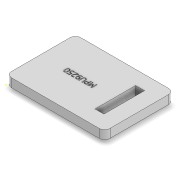
# Autodesk Inventor part: Gyro_box_Top
Saved by Autodesk Inventor 2020 (Build 240168000, 168)
## iProperties
Created: 2019-08-08
Part Number: Gyro_box_Top
Material: Generic
Document SubType Name: Modeling
Designer: chitl
Density: 1 g/cm^3
Appearance: Default
Author: chitl
Autodesk Inventor part; units mm, degrees
ref_plane "YZ Plane" through (0, 0, 0) normal (1, 0, 0) x (0, 1, 0)
ref_plane "XZ Plane" through (0, 0, 0) normal (0, 1, 0) x (-1, 0, 0)
ref_plane "XY Plane" through (0, 0, 0) normal (0, 0, 1) x (1, 0, 0)
sketch "Sketch1" plane through (0, 0, 0) normal (0, 1, 0) x (-1, 0, 0)
  line L0 (0, 0) -> (-56.9976, 0)
  line L1 (-56.9976, 0) -> (-56.9976, -40.1066)
  line L2 (-56.9976, -40.1066) -> (0, -40.1066)
  line L3 (0, -40.1066) -> (0, 0)
  dimension "d0" = 40.1066
  dimension "d1" = 56.9976
  constraints: 8 end point, 2 parallel, 1 horizontal, 1 perpendicular
  measures "d0" distance of L2.end L0.start
  measures "d1" distance between parallel lines of L1 L3
extrude "Extrusion1" add sketch "Sketch1" along normal blind 5
fillet "Fillet1" radius 3.175 2 edges at (0, 2.5, 0) (0, 2.5, -40.1066)
fillet "Fillet2" radius 3.175 2 edges at (56.9976, 2.5, 0) (56.9976, 2.5, -40.1066)
sketch "Sketch2" plane through (0, 0, 0) normal (0, -1, 0) x (1, 0, 0)
  point P0 (0, 0)
sketch "Sketch3" plane through (0, 0, 0) normal (0, -1, 0) x (1, 0, 0)
  arc A0 (53.8226, -40.1066) -> (56.9976, -36.9316) centre (53.8226, -36.9316) ccw projected
  line L0 (56.9976, -3.175) -> (56.9976, -36.9316) projected
  arc A1 (56.9976, -3.175) -> (53.8226, 0) centre (53.8226, -3.175) ccw projected
  line L1 (3.175, 0) -> (53.8226, 0) projected
  arc A2 (3.175, 0) -> (0, -3.175) centre (3.175, -3.175) ccw projected
  line L2 (0, -36.9316) -> (0, -3.175) projected
  arc A3 (0, -36.9316) -> (3.175, -40.1066) centre (3.175, -36.9316) ccw projected
  line L3 (53.8226, -40.1066) -> (3.175, -40.1066) projected
  arc A4 (53.8734, -3.175) -> (53.8226, -3.1242) centre (53.8226, -3.175) ccw
  line L4 (53.8734, -3.175) -> (53.8734, -36.9316)
  arc A5 (53.8226, -36.9824) -> (53.8734, -36.9316) centre (53.8226, -36.9316) ccw
  line L5 (53.8226, -36.9824) -> (3.175, -36.9824)
  arc A6 (3.1242, -36.9316) -> (3.175, -36.9824) centre (3.175, -36.9316) ccw
  line L6 (3.1242, -36.9316) -> (3.1242, -3.175)
  arc A7 (3.175, -3.1242) -> (3.1242, -3.175) centre (3.175, -3.175) ccw
  line L7 (3.175, -3.1242) -> (53.8226, -3.1242)
  point P0 (0, 0)
  dimension "d6" = 3.1242
  constraints: 8 end point, 8 point on circle, 4 centre point, 7 other
  measures "d6" distance between parallel lines of L1 L7
extrude "Extrusion2" add sketch "Sketch3" along normal blind 2 contours L4 A5 L5 A6 L6 A7 L7 A4
sketch "Sketch4" plane through (0, 5, 0) normal (0, 1, 0) x (1, 0, 0)
  line L0 (42.9327, 8.4905) -> (48.1076, 8.4905)
  line L1 (48.1076, 8.4905) -> (48.1076, 31.9976)
  line L2 (48.1076, 31.9976) -> (42.9327, 31.9976)
  line L3 (42.9327, 31.9976) -> (42.9327, 8.4905)
  line L4 (56.9976, 3.175) -> (56.9976, 36.9316) projected
  point P0 (0, 0)
  dimension "d9" = 8.89
  constraints: 8 end point, 2 parallel, 1 horizontal, 1 perpendicular
  measures "d9" distance between parallel lines of L1 L4
extrude "Extrusion3" cut sketch "Sketch4" against normal blind 20.225
sketch "Sketch5" plane through (0, 5, 0) normal (0, 1, 0) x (1, 0, 0)
  line L0 (31.7516, 18.1072) -> (19.4886, 18.1072) construction
  line L1 (19.4886, 18.1072) -> (19.4886, 46.8549) construction
  line L2 (19.4886, 46.8549) -> (31.7516, 46.8549) construction
  line L3 (31.7516, 46.8549) -> (31.7516, 18.1072) construction
  line L4 (28.8296, 21.2194) -> (29.2346, 21.2194)
  line L5 (29.2346, 21.2194) -> (29.2346, 18.5938)
  line L6 (29.2346, 18.5938) -> (30.03, 20.3796)
  line L7 (30.03, 20.3796) -> (30.277, 20.3796)
  line L8 (30.277, 20.3796) -> (31.0649, 18.5938)
  line L9 (31.0649, 18.5938) -> (31.0649, 21.2194)
  line L10 (31.0649, 21.2194) -> (31.4428, 21.2194)
  line L11 (31.4428, 21.2194) -> (31.4428, 18.1714)
  line L12 (31.4428, 18.1714) -> (30.8896, 18.1714)
  line L13 (30.8896, 18.1714) -> (30.1288, 19.8683)
  line L14 (30.1288, 19.8683) -> (29.3927, 18.1714)
  line L15 (29.3927, 18.1714) -> (28.8296, 18.1714)
  line L16 (28.8296, 18.1714) -> (28.8296, 21.2194)
  spline S0 degree 2 poles (26.2855, 19.0903) (26.2855, 19.2879) (26.4262, 19.6436) (26.5522, 19.7671) knots 0 0 0 1 2 2 2
  spline S1 degree 2 poles (26.5522, 19.7671) (26.7103, 19.9227) (27.1376, 20.0832) (27.4636, 20.0832) knots 0 0 0 1 2 2 2
  line L17 (27.4636, 20.0832) -> (27.807, 20.0832)
  line L18 (27.807, 20.0832) -> (27.807, 21.2194)
  line L19 (27.807, 21.2194) -> (28.2121, 21.2194)
  line L20 (28.2121, 21.2194) -> (28.2121, 18.1714)
  line L21 (28.2121, 18.1714) -> (27.4464, 18.1714)
  spline S2 degree 2 poles (27.4464, 18.1714) (27.1747, 18.1714) (26.7943, 18.2604) (26.6485, 18.3616) knots 0 0 0 1 2 2 2
  spline S3 degree 2 poles (26.6485, 18.3616) (26.4781, 18.4777) (26.2855, 18.8359) (26.2855, 19.0903) knots 0 0 0 1 2 2 2
  spline S4 degree 2 poles (26.7078, 19.1026) (26.7078, 18.9445) (26.8165, 18.7124) (26.9277, 18.6383) knots 0 0 0 1 2 2 2
  spline S5 degree 2 poles (26.9277, 18.6383) (27.024, 18.574) (27.2809, 18.5222) (27.4711, 18.5222) knots 0 0 0 1 2 2 2
  line L22 (27.4711, 18.5222) -> (27.807, 18.5222)
  line L23 (27.807, 18.5222) -> (27.807, 19.7374)
  line L24 (27.807, 19.7374) -> (27.5303, 19.7374)
  spline S6 degree 2 poles (27.5303, 19.7374) (27.2833, 19.7374) (26.9795, 19.6584) (26.8807, 19.5546) knots 0 0 0 1 2 2 2
  spline S7 degree 2 poles (26.8807, 19.5546) (26.7893, 19.4633) (26.7078, 19.2484) (26.7078, 19.1026) knots 0 0 0 1 2 2 2
  spline S8 degree 2 poles (24.8356, 21.2837) (25.1048, 21.2837) (25.5049, 21.1429) (25.6457, 21.0021) knots 0 0 0 1 2 2 2
  spline S9 degree 2 poles (25.6457, 21.0021) (25.8063, 20.844) (25.9372, 20.3994) (25.9372, 20.0733) knots 0 0 0 1 2 2 2
  line L25 (25.9372, 20.0733) -> (25.9372, 18.1714)
  line L26 (25.9372, 18.1714) -> (25.5321, 18.1714)
  line L27 (25.5321, 18.1714) -> (25.5321, 20.0733)
  spline S10 degree 2 poles (25.5321, 20.0733) (25.5321, 20.2858) (25.4778, 20.5723) (25.4012, 20.6884) knots 0 0 0 1 2 2 2
  spline S11 degree 2 poles (25.4012, 20.6884) (25.3197, 20.8119) (25.0381, 20.9379) (24.8356, 20.9379) knots 0 0 0 1 2 2 2
  spline S12 degree 2 poles (24.8356, 20.9379) (24.6454, 20.9379) (24.349, 20.8119) (24.2674, 20.6884) knots 0 0 0 1 2 2 2
  spline S13 degree 2 poles (24.2674, 20.6884) (24.1909, 20.5723) (24.1365, 20.2882) (24.1365, 20.0832) knots 0 0 0 1 2 2 2
  line L28 (24.1365, 20.0832) -> (24.1365, 18.1714)
  line L29 (24.1365, 18.1714) -> (23.7315, 18.1714)
  line L30 (23.7315, 18.1714) -> (23.7315, 20.0733)
  spline S14 degree 2 poles (23.7315, 20.0733) (23.7315, 20.392) (23.8599, 20.8465) (24.0229, 21.0021) knots 0 0 0 1 2 2 2
  spline S15 degree 2 poles (24.0229, 21.0021) (24.1686, 21.1453) (24.554, 21.2837) (24.8356, 21.2837) knots 0 0 0 1 2 2 2
  spline S16 degree 2 poles (23.3214, 19.1619) (23.3214, 18.9273) (23.1683, 18.537) (23.0349, 18.3962) knots 0 0 0 1 2 2 2
  spline S17 degree 2 poles (23.0349, 18.3962) (22.9089, 18.2604) (22.5409, 18.1097) (22.3532, 18.1097) knots 0 0 0 1 2 2 2
  spline S18 degree 2 poles (22.3532, 18.1097) (22.1432, 18.1097) (21.8024, 18.2505) (21.6764, 18.3839) knots 0 0 0 1 2 2 2
  spline S19 degree 2 poles (21.6764, 18.3839) (21.5183, 18.5518) (21.3454, 19.0952) (21.3454, 19.5127) knots 0 0 0 1 2 2 2
  spline S20 degree 2 poles (21.3454, 19.5127) (21.3454, 19.8906) (21.5158, 20.5673) (21.6813, 20.7921) knots 0 0 0 1 2 2 2
  spline S21 degree 2 poles (21.6813, 20.7921) (21.8567, 21.0292) (22.3507, 21.2787) (22.7113, 21.2787) knots 0 0 0 1 2 2 2
  spline S22 degree 2 poles (22.7113, 21.2787) (22.7928, 21.2787) (22.9781, 21.2614) (23.0571, 21.2367) knots 0 0 0 1 2 2 2
  line L31 (23.0571, 21.2367) -> (23.0571, 20.844)
  line L32 (23.0571, 20.844) -> (23.0374, 20.844)
  spline S23 degree 2 poles (23.0374, 20.844) (22.9855, 20.8736) (22.7681, 20.9255) (22.657, 20.9255) knots 0 0 0 1 2 2 2
  spline S24 degree 2 poles (22.657, 20.9255) (22.2569, 20.9255) (21.7999, 20.3969) (21.7678, 19.9079) knots 0 0 0 1 2 2 2
  spline S25 degree 2 poles (21.7678, 19.9079) (21.9308, 20.019) (22.2272, 20.1203) (22.4026, 20.1203) knots 0 0 0 1 2 2 2
  spline S26 degree 2 poles (22.4026, 20.1203) (22.5705, 20.1203) (22.8497, 20.0462) (22.9904, 19.94) knots 0 0 0 1 2 2 2
  spline S27 degree 2 poles (22.9904, 19.94) (23.1535, 19.814) (23.3214, 19.4311) (23.3214, 19.1619) knots 0 0 0 1 2 2 2
  spline S28 degree 2 poles (21.7579, 19.4213) (21.7579, 19.1125) (21.8715, 18.7222) (21.9728, 18.616) knots 0 0 0 1 2 2 2
  spline S29 degree 2 poles (21.9728, 18.616) (22.0617, 18.5172) (22.247, 18.4431) (22.3557, 18.4431) knots 0 0 0 1 2 2 2
  spline S30 degree 2 poles (22.3557, 18.4431) (22.6076, 18.4431) (22.9065, 18.8038) (22.9065, 19.1446) knots 0 0 0 1 2 2 2
  spline S31 degree 2 poles (22.9065, 19.1446) (22.9065, 19.3373) (22.8077, 19.5868) (22.699, 19.6757) knots 0 0 0 1 2 2 2
  spline S32 degree 2 poles (22.699, 19.6757) (22.6199, 19.7399) (22.4248, 19.7819) (22.3112, 19.7819) knots 0 0 0 1 2 2 2
  spline S33 degree 2 poles (22.3112, 19.7819) (22.1803, 19.7819) (21.8789, 19.6905) (21.7653, 19.6139) knots 0 0 0 1 2 2 2
  spline S34 degree 2 poles (21.7653, 19.6139) (21.7629, 19.5843) (21.7579, 19.483) (21.7579, 19.4213) knots 0 0 0 1 2 2 2
  line L33 (19.0705, 21.2194) -> (20.9502, 21.2194)
  line L34 (20.9502, 21.2194) -> (20.9502, 20.7872)
  spline S35 degree 2 poles (20.9502, 20.7872) (20.7477, 20.597) (20.3871, 20.2438) (20.2142, 20.0536) knots 0 0 0 1 2 2 2
  spline S36 degree 2 poles (20.2142, 20.0536) (19.8659, 19.6707) (19.6115, 19.2113) (19.6115, 18.9668) knots 0 0 0 1 2 2 2
  spline S37 degree 2 poles (19.6115, 18.9668) (19.6115, 18.8383) (19.6905, 18.6457) (19.7621, 18.5839) knots 0 0 0 1 2 2 2
  spline S38 degree 2 poles (19.7621, 18.5839) (19.8338, 18.5222) (20.0215, 18.4604) (20.1351, 18.4604) knots 0 0 0 1 2 2 2
  spline S39 degree 2 poles (20.1351, 18.4604) (20.2438, 18.4604) (20.4661, 18.5148) (20.5674, 18.5568) knots 0 0 0 1 2 2 2
  spline S40 degree 2 poles (20.5674, 18.5568) (20.6538, 18.5913) (20.8144, 18.6901) (20.8638, 18.7247) knots 0 0 0 1 2 2 2
  line L35 (20.8638, 18.7247) -> (20.886, 18.7247)
  line L36 (20.886, 18.7247) -> (20.886, 18.29)
  spline S41 degree 2 poles (20.886, 18.29) (20.76, 18.2282) (20.308, 18.1072) (20.1055, 18.1072) knots 0 0 0 1 2 2 2
  spline S42 degree 2 poles (20.1055, 18.1072) (19.6782, 18.1072) (19.1965, 18.5592) (19.1965, 18.9445) knots 0 0 0 1 2 2 2
  spline S43 degree 2 poles (19.1965, 18.9445) (19.1965, 19.1249) (19.2805, 19.4262) (19.3546, 19.5546) knots 0 0 0 1 2 2 2
  spline S44 degree 2 poles (19.3546, 19.5546) (19.4287, 19.688) (19.6436, 19.9498) (19.7621, 20.0758) knots 0 0 0 1 2 2 2
  spline S45 degree 2 poles (19.7621, 20.0758) (19.9548, 20.2858) (20.4266, 20.7353) (20.5674, 20.8662) knots 0 0 0 1 2 2 2
  line L37 (20.5674, 20.8662) -> (19.0705, 20.8662)
  line L38 (19.0705, 20.8662) -> (19.0705, 21.2194)
  spline S46 degree 2 poles (16.8154, 20.2512) (16.8154, 20.471) (16.9562, 20.8465) (17.0846, 20.9848) knots 0 0 0 1 2 2 2
  spline S47 degree 2 poles (17.0846, 20.9848) (17.2131, 21.1231) (17.5959, 21.2837) (17.8331, 21.2837) knots 0 0 0 1 2 2 2
  spline S48 degree 2 poles (17.8331, 21.2837) (18.0504, 21.2837) (18.4753, 21.1873) (18.6309, 21.1108) knots 0 0 0 1 2 2 2
  line L39 (18.6309, 21.1108) -> (18.6309, 20.6785)
  line L40 (18.6309, 20.6785) -> (18.6012, 20.6785)
  spline S49 degree 2 poles (18.6012, 20.6785) (18.5543, 20.7131) (18.3789, 20.802) (18.2727, 20.8415) knots 0 0 0 1 2 2 2
  spline S50 degree 2 poles (18.2727, 20.8415) (18.1517, 20.8835) (17.9516, 20.9304) (17.8256, 20.9304) knots 0 0 0 1 2 2 2
  spline S51 degree 2 poles (17.8256, 20.9304) (17.7021, 20.9304) (17.47, 20.8415) (17.386, 20.7452) knots 0 0 0 1 2 2 2
  spline S52 degree 2 poles (17.386, 20.7452) (17.3094, 20.6538) (17.2304, 20.4117) (17.2304, 20.2487) knots 0 0 0 1 2 2 2
  spline S53 degree 2 poles (17.2304, 20.2487) (17.2304, 20.0857) (17.3193, 19.8782) (17.4033, 19.8091) knots 0 0 0 1 2 2 2
  spline S54 degree 2 poles (17.4033, 19.8091) (17.4897, 19.7325) (17.7466, 19.6683) (17.9022, 19.6683) knots 0 0 0 1 2 2 2
  spline S55 degree 2 poles (17.9022, 19.6683) (18.0702, 19.6683) (18.4036, 19.7201) (18.5049, 19.7424) knots 0 0 0 1 2 2 2
  line L41 (18.5049, 19.7424) -> (18.5049, 18.1714)
  line L42 (18.5049, 18.1714) -> (16.8327, 18.1714)
  line L43 (16.8327, 18.1714) -> (16.8327, 18.5296)
  line L44 (16.8327, 18.5296) -> (18.1122, 18.5296)
  line L45 (18.1122, 18.5296) -> (18.1122, 19.3422)
  spline S56 degree 2 poles (18.1122, 19.3422) (18.0381, 19.3323) (17.8948, 19.3249) (17.8355, 19.3249) knots 0 0 0 1 2 2 2
  spline S57 degree 2 poles (17.8355, 19.3249) (17.6009, 19.3249) (17.2773, 19.4015) (17.1291, 19.5151) knots 0 0 0 1 2 2 2
  spline S58 degree 2 poles (17.1291, 19.5151) (16.9784, 19.6287) (16.8154, 19.9745) (16.8154, 20.2512) knots 0 0 0 1 2 2 2
  spline S59 degree 2 poles (14.4788, 19.6954) (14.4788, 20.5155) (14.9555, 21.2837) (15.452, 21.2837) knots 0 0 0 1 2 2 2
  spline S60 degree 2 poles (15.452, 21.2837) (15.9558, 21.2837) (16.4276, 20.5007) (16.4276, 19.6979) knots 0 0 0 1 2 2 2
  spline S61 degree 2 poles (16.4276, 19.6979) (16.4276, 18.8729) (15.9509, 18.1097) (15.452, 18.1097) knots 0 0 0 1 2 2 2
  spline S62 degree 2 poles (15.452, 18.1097) (14.9505, 18.1097) (14.4788, 18.9001) (14.4788, 19.6954) knots 0 0 0 1 2 2 2
  spline S63 degree 2 poles (15.0024, 20.6242) (14.9431, 20.4735) (14.8937, 20.0091) (14.8937, 19.6954) knots 0 0 0 1 2 2 2
  spline S64 degree 2 poles (14.8937, 19.6954) (14.8937, 19.3817) (14.9431, 18.9198) (15.0049, 18.7642) knots 0 0 0 1 2 2 2
  spline S65 degree 2 poles (15.0049, 18.7642) (15.0666, 18.6086) (15.2815, 18.4481) (15.452, 18.4481) knots 0 0 0 1 2 2 2
  spline S66 degree 2 poles (15.452, 18.4481) (15.6224, 18.4481) (15.8422, 18.6086) (15.9064, 18.7692) knots 0 0 0 1 2 2 2
  spline S67 degree 2 poles (15.9064, 18.7692) (15.9682, 18.9248) (16.0127, 19.399) (16.0127, 19.6979) knots 0 0 0 1 2 2 2
  spline S68 degree 2 poles (16.0127, 19.6979) (16.0127, 20.019) (15.9731, 20.4488) (15.9089, 20.6167) knots 0 0 0 1 2 2 2
  spline S69 degree 2 poles (15.9089, 20.6167) (15.8496, 20.7748) (15.6298, 20.9453) (15.452, 20.9453) knots 0 0 0 1 2 2 2
  spline S70 degree 2 poles (15.452, 20.9453) (15.284, 20.9453) (15.0642, 20.7847) (15.0024, 20.6242) knots 0 0 0 1 2 2 2
  point P0 (0, 0)
  constraints: 2 other
emboss "Emboss1" sketch "Sketch5" operation cut depth 1.27 direction (0, -1, 0)
body "Solid1"
